Autodesk Inventor part; units mm, degrees
(part 2 of 2)
  spline S286 degree 2 poles (44.2222, 16.7155) (44.4152, 16.7155) (44.7685, 16.8805) (44.9545, 17.1735) (44.9545, 17.3362) knots 0 0 0 1 2 3 3 3
  spline S287 degree 2 poles (44.9545, 17.3362) (44.9545, 17.5756) (44.5709, 17.915) (44.2432, 17.915) knots 0 0 0 1 2 2 2
  spline S288 degree 2 poles (44.2432, 17.915) (43.927, 17.915) (43.562, 17.5803) (43.562, 17.3222) knots 0 0 0 1 2 2 2
  spline S289 degree 2 poles (43.562, 17.3222) (43.562, 17.0688) (43.927, 16.7155) (44.2222, 16.7155) knots 0 0 0 1 2 2 2
  line L228 (45.2102, 19.8701) -> (44.4803, 19.8701)
  line L229 (44.4803, 19.8701) -> (44.4803, 18.5474)
  line L230 (44.4803, 18.5474) -> (44.1362, 18.5474)
  line L231 (44.1362, 18.5474) -> (42.1602, 19.9375)
  line L232 (42.1602, 19.9375) -> (42.1602, 20.2444)
  line L233 (42.1602, 20.2444) -> (44.1362, 20.2444)
  line L234 (44.1362, 20.2444) -> (44.1362, 20.6558)
  line L235 (44.1362, 20.6558) -> (44.4803, 20.6558)
  line L236 (44.4803, 20.6558) -> (44.4803, 20.2444)
  line L237 (44.4803, 20.2444) -> (45.2102, 20.2444)
  line L238 (45.2102, 20.2444) -> (45.2102, 19.8701)
  line L239 (44.1362, 19.8701) -> (42.76, 19.8701)
  line L240 (42.76, 19.8701) -> (44.1362, 18.9147)
  line L241 (44.1362, 18.9147) -> (44.1362, 19.8701)
  spline S290 degree 2 poles (43.555, 21.6183) (43.469, 21.3835) (43.1529, 21.158) (42.9343, 21.158) knots 0 0 0 1 2 2 2
  spline S291 degree 2 poles (42.9343, 21.158) (42.6019, 21.158) (42.1486, 21.6369) (42.1486, 22.0321) knots 0 0 0 1 2 2 2
  spline S292 degree 2 poles (42.1486, 22.0321) (42.1486, 22.4319) (42.6112, 22.9178) (42.9436, 22.9178) knots 0 0 0 1 2 2 2
  spline S293 degree 2 poles (42.9436, 22.9178) (43.1552, 22.9178) (43.469, 22.6946) (43.555, 22.4668) knots 0 0 0 1 2 2 2
  spline S294 degree 2 poles (43.555, 22.4668) (43.6457, 22.7504) (44.0549, 23.0433) (44.3385, 23.0433) knots 0 0 0 1 2 2 2
  spline S295 degree 2 poles (44.3385, 23.0433) (44.729, 23.0433) (45.2614, 22.49) (45.2614, 22.039) knots 0 0 0 1 2 2 2
  spline S296 degree 2 poles (45.2614, 22.039) (45.2614, 21.5881) (44.7267, 21.0348) (44.3268, 21.0348) knots 0 0 0 1 2 2 2
  spline S297 degree 2 poles (44.3268, 21.0348) (44.0293, 21.0348) (43.6271, 21.337) (43.555, 21.6183) knots 0 0 0 1 2 2 2
  spline S298 degree 2 poles (44.3292, 21.4207) (44.4896, 21.4207) (44.7895, 21.5718) (44.9545, 21.8693) (44.9545, 22.0414) knots 0 0 0 1 2 3 3 3
  spline S299 degree 2 poles (44.9545, 22.0414) (44.9545, 22.311) (44.6081, 22.6574) (44.3431, 22.6574) knots 0 0 0 1 2 2 2
  spline S300 degree 2 poles (44.3431, 22.6574) (44.0711, 22.6574) (43.7178, 22.2994) (43.7178, 22.0297) knots 0 0 0 1 2 2 2
  spline S301 degree 2 poles (43.7178, 22.0297) (43.7178, 21.7647) (44.0665, 21.4207) (44.3292, 21.4207) knots 0 0 0 1 2 2 2
  spline S302 degree 2 poles (42.9204, 21.5439) (43.1366, 21.5439) (43.4109, 21.8205) (43.4109, 22.0414) knots 0 0 0 1 2 2 2
  spline S303 degree 2 poles (43.4109, 22.0414) (43.4109, 22.2576) (43.1389, 22.5319) (42.9413, 22.5319) knots 0 0 0 1 2 2 2
  spline S304 degree 2 poles (42.9413, 22.5319) (42.7367, 22.5319) (42.4555, 22.2506) (42.4555, 22.039) knots 0 0 0 1 2 2 2
  spline S305 degree 2 poles (42.4555, 22.039) (42.4555, 21.8228) (42.7298, 21.5439) (42.9204, 21.5439) knots 0 0 0 1 2 2 2
  point P0 (0, 0)
  constraints: 2 other
extrude "Wyciągnięcie proste5" cut sketch "Szkic8" against normal blind 1
